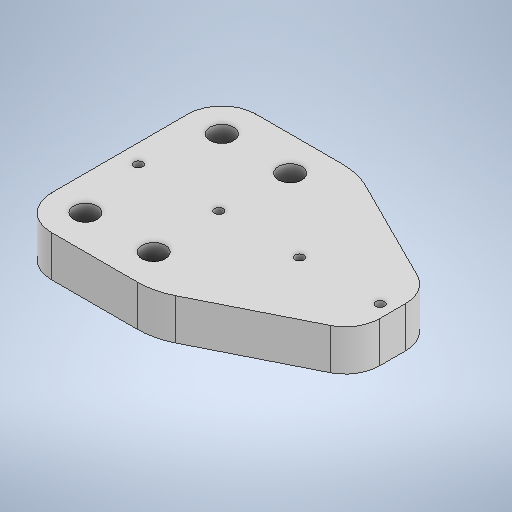
# Autodesk Inventor part: Linear_Mount
Saved by Autodesk Inventor 2025.1 (Build 291241020, 241B)
## iProperties
Created: 2024-11-27
Part Number: Linear_Mount
Material: Generic
Document SubType Name: Modeling
Designer: AtuStem
Density: 1 g/cm^3
Appearance: Default
Author: AtuStem
Autodesk Inventor part; units mm, degrees
ref_plane "YZ Plane" through (0, 0, 0) normal (1, 0, 0) x (0, 1, 0)
ref_plane "XZ Plane" through (0, 0, 0) normal (0, 1, 0) x (-1, 0, 0)
ref_plane "XY Plane" through (0, 0, 0) normal (0, 0, 1) x (1, 0, 0)
sketch "Sketch1" plane through (0, 0, 0) normal (0, 1, 0) x (-1, 0, 0)
  circle A0 centre (21.9, 0) radius 0.8
  circle A1 centre (6.9, 0) radius 0.8
  circle A2 centre (-8.1, 0) radius 0.8
  circle A3 centre (-23.1, 0) radius 0.8
  line L0 (25.4, -19.05) -> (-25.4, -19.05)
  line L1 (-25.4, 19.05) -> (-25.4, -19.05)
  line L2 (-25.4, 19.05) -> (25.4, 19.05)
  line L3 (25.4, -19.05) -> (25.4, 19.05)
  circle A4 centre (19.05, -12.7) radius 2.1844
  circle A5 centre (6.35, -12.7) radius 2.1844
  circle A6 centre (6.35, 12.7) radius 2.1844
  circle A7 centre (19.05, 12.7) radius 2.1844
  line L4 (25.4, 0) -> (-25.4, 0)
  line L5 (0, -19.05) -> (0, 19.05)
  circle A8 centre (0, 0) radius 1.235
  line L6 (-25.4, 0) -> (-25.4, 6.35)
  line L7 (-25.4, 6.35) -> (-25.4, -6.35)
  line L8 (0, 19.05) -> (-25.4, 6.35)
  line L9 (-25.4, -6.35) -> (0, -19.05)
  point P0 (21.9, 0)
  dimension "d3" = 1.6
  dimension "d4" = 1.6
  dimension "d5" = 1.6
  dimension "d6" = 1.6
  dimension "d7" = 6.35
  dimension "d8" = 12.7
  constraints: 20 end point, 9 centre point, 5 midpoint, 2 point on line
  measures "d3" diameter of A0
  measures "d4" diameter of A1
  measures "d5" diameter of A2
  measures "d6" diameter of A3
  measures "d7" distance of L4.end L6.end
  measures "d8" distance of L6.end L7.end
extrude "Extrusion1" add sketch "Sketch1" along normal blind 7.62 contours L4 L3 L0 L5 A8 A1 A0 | A0 L4 A1 A8 L5 L2 L3 | L9 L1 L4 A3 A2 A8 L5 | L5 A8 L4 A2 A3 L1 L8 | A8 L5 L4 | L4 L5 A8 | A8 L4 L5 | L5 L4 A8
fillet "Fillet1" radius 6.35 2 edges at (-25.4, 3.81, 19.05) (-25.4, 3.81, -19.05)
fillet "Fillet2" radius 6.35 2 edges at (25.4, 3.81, -6.35) (25.4, 3.81, 6.35)
fillet "Fillet3" radius 12.7 2 edges at (0, 3.81, -19.05) (0, 3.81, 19.05)
body "Solid1"
